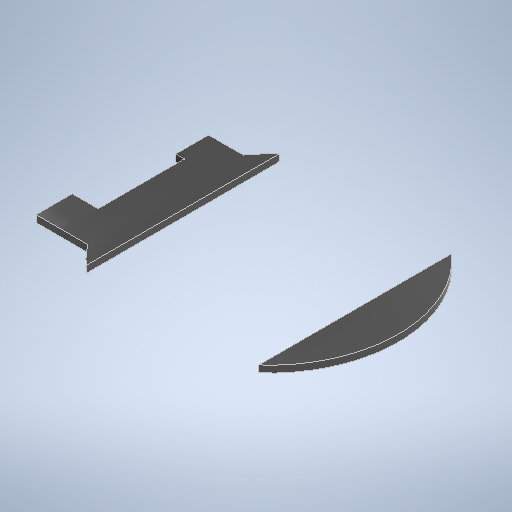
# Autodesk Inventor part: Soportes
Saved by Autodesk Inventor 2025.2 (Build 292293000, 293)
## iProperties
Created: 2025-11-06
Part Number: Soportes
Material: Genérico
Document SubType Name: Modeling
Designer: Dax
Density: 1 g/cm^3
Appearance: Gris oscuro
Author: Dax
Autodesk Inventor part; units mm, degrees
ref_plane "YZ Plane" through (0, 0, 0) normal (1, 0, 0) x (0, 1, 0)
ref_plane "XZ Plane" through (0, 0, 0) normal (0, 1, 0) x (-1, 0, 0)
ref_plane "XY Plane" through (0, 0, 0) normal (0, 0, 1) x (1, 0, 0)
sketch "Boceto1" plane through (0, 0, 0) normal (0, 1, 0) x (-1, 0, 0)
  line L0 (-50, 0) -> (-50, -55.9017)
  line L1 (-50, 0) -> (-50, 55.9017)
  line L2 (50, 0) -> (50, -55.9017)
  line L3 (50, 0) -> (50, 55.9017)
  line L4 (50, 0) -> (50, -45)
  line L5 (60, -45) -> (80, -45)
  line L6 (80, -45) -> (80, -26)
  line L7 (80, -26) -> (75, -26)
  line L8 (50, 0) -> (50, 45)
  line L9 (60, 45) -> (90, 45)
  line L10 (90, 45) -> (90, 24)
  line L11 (90, 24) -> (75, 24)
  line L12 (75, -26) -> (75, 24)
  arc A0 (50, -55.9017) -> (60, -45) centre (0, 0) ccw
  arc A1 (60, 45) -> (50, 55.9017) centre (0, 0) ccw
  arc A2 (-50, 55.9017) -> (-50, -55.9017) centre (0, 0) ccw
  dimension "d2" = 45
  dimension "d3" = 30
  dimension "d4" = 19
  dimension "d5" = 5
  dimension "d6" = 45
  dimension "d7" = 40
  dimension "d8" = 21
  constraints: 26 end point, 7 perpendicular, 6 point on circle, 3 centre point, 2 point on line, 1 coincident, 1 vertical
  measures "d2" distance of L2.start L4.end
  measures "d3" distance of L4.end L5.end
  measures "d4" distance of L5.end L6.end
  measures "d5" distance of L6.end L7.end
  measures "d6" distance of L2.start L8.end
  measures "d7" distance of L8.end L9.end
  measures "d8" distance of L9.end L10.end
extrude "Extrusión1" add sketch "Boceto1" along normal blind 4
